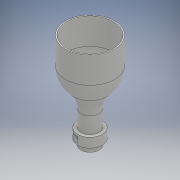
# Autodesk Inventor part: Outer tube
Saved by Autodesk Inventor 2018.3 (Build 223284000, 284)
## iProperties
Created: 2020-03-27
Part Number: Outer tube
Material: Generic
Document SubType Name: Modeling
Designer: ToreDenStore
Density: 1 g/cm^3
Appearance: Default
Author: ToreDenStore
Autodesk Inventor part; units mm, degrees
ref_plane "YZ Plane" through (0, 0, 0) normal (1, 0, 0) x (0, 1, 0)
ref_plane "XZ Plane" through (0, 0, 0) normal (0, 1, 0) x (-1, 0, 0)
ref_plane "XY Plane" through (0, 0, 0) normal (0, 0, 1) x (1, 0, 0)
sketch "Sketch2" plane through (0, 0, 0) normal (1, 0, 0) x (0, 1, 0)
  line L0 (0, 0) -> (0, -50)
  arc A0 (-14.6447, -85.3553) -> (0, -50) centre (-50, -50) ccw
  line L1 (-50, -50) -> (-14.6447, -85.3553) construction
  line L2 (-50, -50) -> (0, -50) construction
  arc A1 (-14.6447, -85.3553) -> (-29.2893, -120.7107) centre (20.7107, -120.7107) ccw
  line L3 (20.7107, -120.7107) -> (-29.2893, -120.7107) construction
  line L4 (20.7107, -120.7107) -> (-14.6447, -85.3553) construction
  line L5 (-29.2893, -120.7107) -> (-29.2893, -140.7107)
  line L6 (0, 0) -> (-92.5786, 0) construction
  line L7 (-2, 0) -> (-2, -50)
  arc A2 (-16.6447, -85.3553) -> (-2, -50) centre (-52, -50) ccw
  arc A3 (-16.6447, -85.3553) -> (-31.2893, -120.7107) centre (18.7107, -120.7107) ccw
  line L8 (-31.2893, -120.7107) -> (-31.2893, -140.7107)
  line L9 (0, 0) -> (-2, 0)
  line L10 (-29.2893, -140.7107) -> (-31.2893, -140.7107)
  line L11 (-46.2893, -140.7107) -> (-46.2893, 0)
  line L12 (-31.2893, -140.7107) -> (-46.2893, -140.7107) construction
  dimension "d18" = 50
  dimension "d19" = 45
  dimension "d20" = 45
  dimension "d21" = 50
  dimension "d22" = 50
  dimension "d23" = 20
  dimension "d26" = 2
  dimension "d31" = 90
  dimension "d32" = 15
  constraints: 26 end point, 8 point on circle, 4 centre point, 4 horizontal, 2 tangent, 2 vertical, 1 collinear, 1 midpoint, 11 other
  measures "d18" distance of L0.start L0.end
  measures "d19" angle of L1 L2
  measures "d20" angle of L4 L3
  measures "d21" radius of A0
  measures "d22" radius of A1
  measures "d23" distance of L3.end L5.end
  measures "d26" distance of L0.start L7.start
  measures "d31" angle of L12 L11
  measures "d32" distance of L8.end L11.start
revolve "Revolution1" add sketch "Sketch2" angle 360 about axis through (0, -46.2893, -140.7107) along (0, 0, 1)
sketch "Sketch3" plane through (0, -46.2893, -140.7107) normal (0, 0, -1) x (-1, 0, 0)
  circle A0 centre (0, 0) radius 15 projected
  circle A1 centre (0, 0) radius 2
  circle A2 centre (0, 0) radius 4
  point P0 (0, 46.2893)
  dimension "d34" = 4
  dimension "d35" = 8
  constraints: 2 centre point, 2 coincident
  measures "d34" diameter of A1
  measures "d35" diameter of A2
extrude "Extrusion1" add sketch "Sketch3" against normal blind 10 contours A2
sketch "Sketch4" plane through (0, -46.2893, -140.7107) normal (0, 0, -1) x (-1, 0, 0)
  circle A0 centre (0, 0) radius 15 projected
  circle A1 centre (0, 0) radius 4 projected
  line L0 (-3.873, -1) -> (-14.9666, -1)
  line L1 (-3.873, 1) -> (-14.9666, 1)
  circle A2 centre (0, 0) radius 15 projected
  line L2 (-4, 0) -> (-15, 0) construction
  line L3 (64.8051, 46.2893) -> (-64.8051, 46.2893) projected
  point P0 (0, 46.2893)
  dimension "d38" = 0
  dimension "d39" = 1
  dimension "d40" = 1
  constraints: 6 end point, 5 point on circle, 2 horizontal, 2 parallel, 2 other
  measures "d38" distance from line of A1.centre L2
  measures "d39" distance between parallel lines of L0 L2
  measures "d40" distance between parallel lines of L1 L2
extrude "Extrusion2" add sketch "Sketch4" against normal blind 4 contours L1 A1 L0 A0 picked at (-7.656, -0.1112)
pattern_circular "Circular Pattern1" count 5 over 360 about axis through (0, -46.2893, -140.7107) along (0, 0, 1) of "Extrusion2"
sketch "Sketch5" plane through (0, -46.2893, -140.7107) normal (0, 0, -1) x (-1, 0, 0)
  circle A0 centre (0, 0) radius 17 projected
  circle A1 centre (0, 0) radius 15
  point P0 (0, 46.2893)
  dimension "d46" = 30
  constraints: 1 centre point, 1 coincident
  measures "d46" diameter of A1
extrude "Extrusion3" add sketch "Sketch5" along normal blind 15
sketch "Sketch6" plane through (0, -46.2893, -155.7107) normal (0, 0, -1) x (-1, 0, 0)
  circle A0 centre (0, 0) radius 17 projected
  circle A1 centre (0, 0) radius 23
  point P0 (0, 46.2893)
  dimension "d49" = 46
  constraints: 1 centre point, 1 coincident
  measures "d49" diameter of A1
extrude "Extrusion4" add sketch "Sketch6" against normal blind 4
sketch "Sketch7" plane through (0, -46.2893, -155.7107) normal (0, 0, -1) x (-1, 0, 0)
  circle A0 centre (0, 0) radius 23 projected
  circle A1 centre (0, 0) radius 21
  point P0 (0, 46.2893)
  dimension "d52" = 42
  constraints: 1 centre point, 1 coincident
  measures "d52" diameter of A1
extrude "Extrusion5" add sketch "Sketch7" along normal blind 10
sketch "Sketch8" plane through (0, -46.2893, -165.7107) normal (0, 0, -1) x (-1, 0, 0)
  circle A0 centre (0, 0) radius 21 projected
  circle A1 centre (0, 0) radius 23 projected
  circle A2 centre (0, 0) radius 23 projected
  line L0 (0, -23) -> (0, -21)
  line L1 (23, 0) -> (21, 0)
  line L2 (64.8051, 46.2893) -> (-64.8051, 46.2893) projected
  line L3 (0, -64.8051) -> (0, 64.8051) projected
  point P0 (0, 46.2893)
  dimension "d55" = 2
  dimension "d56" = 2
  constraints: 4 end point, 4 point on circle, 1 collinear, 1 parallel, 1 perpendicular, 1 vertical
  measures "d55" distance of L1.start L1.end
  measures "d56" distance of L0.start L0.end
extrude "Extrusion6" cut sketch "Sketch8" against normal blind 10 contours A0 L1 A1 L0
ref_plane "Mirror plane" through (14.9666, -47.2893, -153.2107) normal (0, 0, -1) x (-1, 0, 0)
mirror "Mirror1" about plane through (14.9666, -47.2893, -153.2107) normal (0, 0, -1) of "Extrusion2", "Circular Pattern1", "Extrusion1"
ref_plane "Mirror plane 2" through (0, -46.2893, -160.7107) normal (0, 0, -1) x (-1, 0, 0)
mirror "Mirror2" about plane through (0, -46.2893, -160.7107) normal (0, 0, -1) of "Extrusion4", "Extrusion3"
equation "\"d40\" = d39"
body "Solid1"
